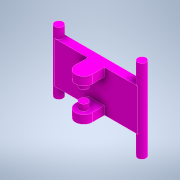
# Autodesk Inventor part: enEffector
Saved by Autodesk Inventor 2022 (Build 260153000, 153)
## iProperties
Created: 2021-12-27
Part Number: enEffector
Material: Generic
Document SubType Name: Modeling
Designer: G S SHOURIE
Density: 1 g/cm^3
Appearance: Magenta
Author: G S SHOURIE
Autodesk Inventor part; units mm, degrees
ref_plane "YZ Plane" through (0, 0, 0) normal (1, 0, 0) x (0, 1, 0)
ref_plane "XZ Plane" through (0, 0, 0) normal (0, 1, 0) x (-1, 0, 0)
ref_plane "XY Plane" through (0, 0, 0) normal (0, 0, 1) x (1, 0, 0)
sketch "Sketch1" plane through (0, 0, 0) normal (0, 0, 1) x (1, 0, 0)
  line L0 (-50, 25) -> (50, 25)
  line L1 (50, 25) -> (50, -25)
  line L2 (50, -25) -> (-50, -25)
  line L3 (-50, -25) -> (-50, 25)
  point P0 (0, 0)
  dimension "d0" = 100
  dimension "d1" = 50
  dimension "d2" = 25
  dimension "d3" = 50
  constraints: 8 end point, 2 parallel, 1 horizontal, 1 perpendicular
  measures "d0" distance of L1.end L2.end
  measures "d1" distance of L0.end L1.end
  measures "d2" distance from line of L0 point (0, 0)
  measures "d3" distance from line of L3 point (0, 0)
extrude "Extrusion1" add sketch "Sketch1" along normal mid plane 10
sketch "Sketch3" plane through (0, 0, 0) normal (0, 1, 0) x (-1, 0, 0)
  line L0 (50, -5) -> (50, 5) projected
  circle A0 centre (50, 0) radius 5
  line L1 (-50, -5) -> (-50, 5) projected
  point P0 (0, 0)
  constraints: 1 midpoint, 1 vertical alignment, 2 other
extrude "Extrusion2" add sketch "Sketch3" along normal mid plane 75
sketch "Sketch4" plane through (0, 0, 0) normal (0, 1, 0) x (-1, 0, 0)
  line L0 (-50, -5) -> (-50, 5) projected
  circle A0 centre (-50, 0) radius 5
  point P0 (0, 0)
  constraints: 1 midpoint, 1 vertical alignment, 2 other
extrude "Extrusion3" add sketch "Sketch4" along normal mid plane 100
sketch "Sketch8" plane through (-50, 25, 0) normal (0, 1, 0) x (1, 0, 0)
  line L0 (60, 0) -> (40, 0)
  line L1 (40, 0) -> (40, -20)
  line L2 (40, -20) -> (60, -20)
  line L3 (60, -20) -> (60, 0)
  arc A0 (40, -20) -> (60, -20) centre (50, -20) ccw
  point P0 (50, 0)
  dimension "d16" = 20
  dimension "d17" = 20
  dimension "d18" = 10
  constraints: 8 end point, 2 parallel, 2 point on circle, 1 centre point, 1 horizontal, 1 midpoint, 1 perpendicular, 1 tangent
  measures "d16" distance of L2.end L1.end
  measures "d17" distance of L1.end L0.end
  measures "d18" distance from line of L1 point (50, 0)
extrude "Extrusion6" add sketch "Sketch8" against normal blind 10
mirror "Mirror1" about plane through (0, 0, 0) normal (0, 1, 0) of "Extrusion6"
sketch "Sketch9" plane through (-50, 15, 0) normal (0, -1, 0) x (1, 0, 0)
  arc A0 (60, 20) -> (40, 20) centre (50, 20) ccw projected
  circle A1 centre (50, 20) radius 5
  point P0 (50, 0)
  dimension "d21" = 10
  constraints: 1 centre point, 1 coincident
  measures "d21" diameter of A1
extrude "Extrusion7" add sketch "Sketch9" along normal blind 7.5
mirror "Mirror2" about plane through (0, 0, 0) normal (0, 1, 0) of "Extrusion7"
body "Solid1"
